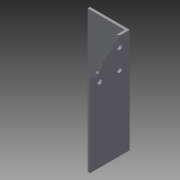
# Autodesk Inventor part: 2x2 angle vertical right
Saved by Autodesk Inventor 2015 SP1 (Build 190203100, 203)
## iProperties
Created: 2015-01-15
Part Number: 2x2 angle vertical right
Material: Generic
Document SubType Name: Modeling
Designer: Jarod
Density: 1 g/cm^3
Appearance: Default
Author: Jarod
Autodesk Inventor part; units mm, degrees
ref_plane "YZ Plane" through (0, 0, 0) normal (1, 0, 0) x (0, 1, 0)
ref_plane "XZ Plane" through (0, 0, 0) normal (0, 1, 0) x (-1, 0, 0)
ref_plane "XY Plane" through (0, 0, 0) normal (0, 0, 1) x (1, 0, 0)
sketch "Sketch1" plane through (0, 0, 0) normal (0, 1, 0) x (-1, 0, 0)
  line L0 (0, 0) -> (3.175, 0)
  line L1 (3.175, 0) -> (3.175, 50.8)
  line L2 (3.175, 50.8) -> (0, 50.8)
  line L3 (0, 50.8) -> (0, 0)
  line L4 (0, 0) -> (50.8, 0)
  line L5 (50.8, 0) -> (50.8, 3.175)
  line L6 (50.8, 3.175) -> (0, 3.175)
  line L7 (0, 3.175) -> (0, 0)
  dimension "d0" = 3.175
  dimension "d1" = 50.8
  dimension "d2" = 50.8
  dimension "d3" = 3.175
  constraints: 16 end point, 4 parallel, 2 horizontal, 2 perpendicular
  measures "d0" distance of L2.end L1.end
  measures "d1" distance of L1.end L0.end
  measures "d2" distance of L6.end L5.end
  measures "d3" distance of L5.end L4.end
extrude "Extrusion1" add sketch "Sketch1" along normal blind 133.35
sketch "Sketch2" plane through (0, 0, 50.8) normal (1, 0, 0) x (0, 0, -1)
  line L0 (0, 0) -> (50.8, 0) projected
  line L1 (50.8, 0) -> (50.8, 133.35) projected
  line L2 (0, 133.35) -> (50.8, 133.35) projected
  line L3 (0, 0) -> (0, 133.35) projected
  point P0 (12.7, 120.65)
  point P1 (38.1, 120.65)
  point P2 (38.1, 95.25)
  point P3 (12.7, 95.25)
  dimension "d6" = 12.7
  dimension "d7" = 12.7
  dimension "d8" = 12.7
  dimension "d9" = 12.7
  dimension "d10" = 12.7
  dimension "d11" = 12.7
  dimension "d12" = 38.1
  dimension "d13" = 38.1
  measures "d6" distance from line of L3 point (12.7, 120.65)
  measures "d7" distance from line of L2 point (12.7, 120.65)
  measures "d8" distance from line of L2 point (38.1, 120.65)
  measures "d9" distance from line of L1 point (38.1, 120.65)
  measures "d10" distance from line of L1 point (38.1, 95.25)
  measures "d11" distance from line of L3 point (12.7, 95.25)
  measures "d12" distance from line of L2 point (12.7, 95.25)
  measures "d13" distance from line of point (38.1, 95.25) L2
hole "Hole1" at (0, 120.65, 38.1) at (0, 120.65, 12.7) at (0, 95.25, 12.7) at (0, 95.25, 38.1) direction (-1, 0, 0) diameter 6.35 end through all
sketch "Sketch3" plane through (0, 0, 0) normal (0, 0, -1) x (-1, 0, 0)
  line L0 (0, 133.35) -> (50.8, 133.35) projected
  line L1 (0, 0) -> (0, 133.35) projected
  line L2 (0, 0) -> (50.8, 0) projected
  line L3 (50.8, 0) -> (50.8, 133.35) projected
  point P0 (12.7, 69.85)
  point P1 (38.1, 69.85)
  point P2 (38.1, 44.45)
  point P3 (12.7, 44.45)
  dimension "d21" = 12.7
  dimension "d22" = 12.7
  dimension "d23" = 63.5
  dimension "d24" = 63.5
  dimension "d32" = 88.9
  dimension "d33" = 88.9
  dimension "d34" = 12.7
  dimension "d35" = 12.7
  measures "d21" distance from line of L1 point (12.7, 69.85)
  measures "d22" distance from line of L3 point (38.1, 69.85)
  measures "d23" distance from line of L0 point (12.7, 69.85)
  measures "d24" distance from line of L0 point (38.1, 69.85)
  measures "d32" distance from line of point (12.7, 44.45) L0
  measures "d33" distance from line of point (38.1, 44.45) L0
  measures "d34" distance from line of L3 point (38.1, 44.45)
  measures "d35" distance from line of L1 point (12.7, 44.45)
hole "Hole3" at (-12.7, 69.85, 0) at (-38.1, 69.85, 0) at (-38.1, 44.45, 0) at (-12.7, 44.45, 0) direction (0, 0, 1) diameter 6.35 end through all
body "Solid1"
